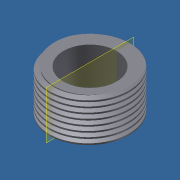
# Autodesk Inventor part: LUVA COM ROSCA TRAPEZOIDAL
Saved by Autodesk Inventor 2012 SP2 (Build 160219200, 219)
## iProperties
Created: 2012-07-24
Part Number: LUVA COM ROSCA TRAPEZOIDAL
Material: Carbon Steel
Document SubType Name: Modeling
Designer: bruno.silveira
Mass: 689.809 g
Surface Area: 114.982 cm^2
Volume: 87.6504 cm^3
Density: 7.87 g/cm^3
Author: bruno.silveira
Autodesk Inventor part; units mm, degrees
ref_plane "YZ Plane" through (0, 0, 0) normal (1, 0, 0) x (0, 1, 0)
ref_plane "XZ Plane" through (0, 0, 0) normal (0, 1, 0) x (-1, 0, 0)
ref_plane "XY Plane" through (0, 0, 0) normal (0, 0, 1) x (1, 0, 0)
sketch "Sketch1" plane through (0, 0, 0) normal (0, 0, 1) x (1, 0, 0)
  circle A0 centre (0, 0) radius 30
  dimension "d0" = 60
  constraints: 1 centre point, 1 coincident
  measures "d0" diameter of A0
extrude "Extrusion1" add sketch "Sketch1" along normal blind 31
sketch "Sketch2" plane through (0, 0, 31) normal (0, 0, 1) x (1, 0, 0)
  circle A0 centre (0, 0) radius 30 projected
  circle A1 centre (0, 0) radius 20
  dimension "d3" = 40
  constraints: 1 centre point, 1 coincident
  measures "d3" diameter of A1
extrude "Extrusion2" cut sketch "Sketch2" against normal blind 31 contours A1
sketch "Sketch3" plane through (0, 0, 0) normal (0, 0, -1) x (-1, 0, 0)
  circle A0 centre (0, 0) radius 20 projected
  circle A1 centre (0, 0) radius 30 projected
  circle A2 centre (0, 0) radius 25
  dimension "d6" = 50
  constraints: 1 centre point, 1 coincident
  measures "d6" diameter of A2
extrude "Extrusion3" cut sketch "Sketch3" against normal blind 3 contours A2
sketch "Sketch4" plane through (0, 0, 0) normal (1, 0, 0) x (0, 1, 0)
  line L0 (-30, 31) -> (30, 31) projected
  line L1 (-30, 0) -> (30, 0) projected
  line L2 (26.5, 33.3397) -> (26.5, 32.3397)
  line L3 (26.5, 32.3397) -> (30.5, 31.2679)
  line L4 (30.5, 31.2679) -> (30.5, 34.4115)
  line L5 (30.5, 34.4115) -> (26.5, 33.3397)
  line L6 (0, 0) -> (0, 31)
  line L7 (26.5, 32.8397) -> (30.5, 32.8397)
  dimension "d9" = 53
  dimension "d10" = 4
  dimension "d11" = 30
  dimension "d12" = 15
  dimension "d13" = 1
  constraints: 12 end point, 3 midpoint, 2 perpendicular, 1 parallel
  measures "d9" diameter of L2 L6
  measures "d10" distance between parallel lines of L4 L2
  measures "d11" angle of L3 L5
  measures "d12" angle of L7 L5
  measures "d13" distance of L2.start L2.end
coil "Coil1" sketch "Sketch4" operation cut axis through (0, 0, 0) along (0, 0, -1) pitch 4 turns 9 hand right
body "Solid1"
